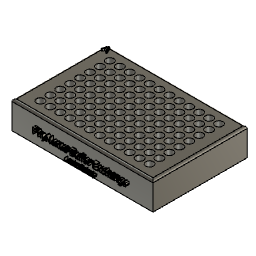
PhyNexus_Adapter v4 (Autodesk Fusion 360 design; units mm, degrees)
Autodesk Fusion 360 part; units mm, degrees
sketch "Sketch1" plane through (0, 0, 0) normal (0, 0, 1) x (1, 0, 0)
  line L0 (0, 0) -> (-127.8, 0)
  line L1 (-127.8, 0) -> (-127.8, 85.5)
  line L2 (-127.8, 85.5) -> (0, 85.5)
  line L3 (0, 85.5) -> (0, 0)
  dimension "d1" = 127.8
  dimension "d2" = 85.5
  constraint horizontal L0
  constraint vertical L1
  constraint horizontal L2
  constraint vertical L3
  constraint coincident L0.start L3.end
  measures "d1" distance of L0.start L0.end
  measures "d2" distance of L0.start L2.end
extrude "Extrude1" add sketch "Sketch1" along normal blind 25
sketch "Sketch2" plane through (0, 0, 25) normal (0, 0, 1) x (-1, 0, 0)
  line L0 (0, -85.5) -> (127.8, -85.5)
  line L1 (127.8, -85.5) -> (127.8, 0)
  line L2 (127.8, 0) -> (0, 0)
  line L3 (0, 0) -> (0, -85.5)
  circle A0 centre (113.4, -74.3) radius 3.5
  circle A1 centre (104.4, -74.3) radius 3.5
  circle A2 centre (95.4, -74.3) radius 3.5
  circle A3 centre (86.4, -74.3) radius 3.5
  circle A4 centre (77.4, -74.3) radius 3.5
  circle A5 centre (68.4, -74.3) radius 3.5
  circle A6 centre (59.4, -74.3) radius 3.5
  circle A7 centre (50.4, -74.3) radius 3.5
  circle A8 centre (41.4, -74.3) radius 3.5
  circle A9 centre (32.4, -74.3) radius 3.5
  circle A10 centre (23.4, -74.3) radius 3.5
  circle A11 centre (14.4, -74.3) radius 3.5
  circle A12 centre (113.4, -65.3) radius 3.5
  circle A13 centre (104.4, -65.3) radius 3.5
  circle A14 centre (95.4, -65.3) radius 3.5
  circle A15 centre (86.4, -65.3) radius 3.5
  circle A16 centre (77.4, -65.3) radius 3.5
  circle A17 centre (68.4, -65.3) radius 3.5
  circle A18 centre (59.4, -65.3) radius 3.5
  circle A19 centre (50.4, -65.3) radius 3.5
  circle A20 centre (41.4, -65.3) radius 3.5
  circle A21 centre (32.4, -65.3) radius 3.5
  circle A22 centre (23.4, -65.3) radius 3.5
  circle A23 centre (14.4, -65.3) radius 3.5
  circle A24 centre (113.4, -56.3) radius 3.5
  circle A25 centre (104.4, -56.3) radius 3.5
  circle A26 centre (95.4, -56.3) radius 3.5
  circle A27 centre (86.4, -56.3) radius 3.5
  circle A28 centre (77.4, -56.3) radius 3.5
  circle A29 centre (68.4, -56.3) radius 3.5
  circle A30 centre (59.4, -56.3) radius 3.5
  circle A31 centre (50.4, -56.3) radius 3.5
  circle A32 centre (41.4, -56.3) radius 3.5
  circle A33 centre (32.4, -56.3) radius 3.5
  circle A34 centre (23.4, -56.3) radius 3.5
  circle A35 centre (14.4, -56.3) radius 3.5
  circle A36 centre (113.4, -47.3) radius 3.5
  circle A37 centre (104.4, -47.3) radius 3.5
  circle A38 centre (95.4, -47.3) radius 3.5
  circle A39 centre (86.4, -47.3) radius 3.5
  circle A40 centre (77.4, -47.3) radius 3.5
  circle A41 centre (68.4, -47.3) radius 3.5
  circle A42 centre (59.4, -47.3) radius 3.5
  circle A43 centre (50.4, -47.3) radius 3.5
  circle A44 centre (41.4, -47.3) radius 3.5
  circle A45 centre (32.4, -47.3) radius 3.5
  circle A46 centre (23.4, -47.3) radius 3.5
  circle A47 centre (14.4, -47.3) radius 3.5
  circle A48 centre (113.4, -38.3) radius 3.5
  circle A49 centre (104.4, -38.3) radius 3.5
  circle A50 centre (95.4, -38.3) radius 3.5
  circle A51 centre (86.4, -38.3) radius 3.5
  circle A52 centre (77.4, -38.3) radius 3.5
  circle A53 centre (68.4, -38.3) radius 3.5
  circle A54 centre (59.4, -38.3) radius 3.5
  circle A55 centre (50.4, -38.3) radius 3.5
  circle A56 centre (41.4, -38.3) radius 3.5
  circle A57 centre (32.4, -38.3) radius 3.5
  circle A58 centre (23.4, -38.3) radius 3.5
  circle A59 centre (14.4, -38.3) radius 3.5
  circle A60 centre (113.4, -29.3) radius 3.5
  circle A61 centre (104.4, -29.3) radius 3.5
  circle A62 centre (95.4, -29.3) radius 3.5
  circle A63 centre (86.4, -29.3) radius 3.5
  circle A64 centre (77.4, -29.3) radius 3.5
  circle A65 centre (68.4, -29.3) radius 3.5
  circle A66 centre (59.4, -29.3) radius 3.5
  circle A67 centre (50.4, -29.3) radius 3.5
  circle A68 centre (41.4, -29.3) radius 3.5
  circle A69 centre (32.4, -29.3) radius 3.5
  circle A70 centre (23.4, -29.3) radius 3.5
  circle A71 centre (14.4, -29.3) radius 3.5
  circle A72 centre (113.4, -20.3) radius 3.5
  circle A73 centre (104.4, -20.3) radius 3.5
  circle A74 centre (95.4, -20.3) radius 3.5
  circle A75 centre (86.4, -20.3) radius 3.5
  circle A76 centre (77.4, -20.3) radius 3.5
  circle A77 centre (68.4, -20.3) radius 3.5
  circle A78 centre (59.4, -20.3) radius 3.5
  circle A79 centre (50.4, -20.3) radius 3.5
  circle A80 centre (41.4, -20.3) radius 3.5
  circle A81 centre (32.4, -20.3) radius 3.5
  circle A82 centre (23.4, -20.3) radius 3.5
  circle A83 centre (14.4, -20.3) radius 3.5
  circle A84 centre (113.4, -11.3) radius 3.5
  circle A85 centre (104.4, -11.3) radius 3.5
  circle A86 centre (95.4, -11.3) radius 3.5
  circle A87 centre (86.4, -11.3) radius 3.5
  circle A88 centre (77.4, -11.3) radius 3.5
  circle A89 centre (68.4, -11.3) radius 3.5
  circle A90 centre (59.4, -11.3) radius 3.5
  circle A91 centre (50.4, -11.3) radius 3.5
  circle A92 centre (41.4, -11.3) radius 3.5
  circle A93 centre (32.4, -11.3) radius 3.5
  circle A94 centre (23.4, -11.3) radius 3.5
  circle A95 centre (14.4, -11.3) radius 3.5
  dimension "d15" = 7
  dimension "d18" = -9
  dimension "d19" = 9
  measures "d15" diameter of A0
extrude "Extrude2" cut sketch "Sketch2" against normal blind 40 contours A0 | A1 | A2 | A3 | A4 | A5 | A6 | A7 | A8 | A9 | A10 | A11 | A12 | A13 | A14 | A15 | A16 | A17 | A18 | A19 | A20 | A21 | A22 | A23 | A24 | A25 | A26 | A27 | A28 | A29 | A30 | A31 | A32 | A33 | A34 | A35 | A36 | A37 | A38 | A39 | A40 | A41 | A42 | A43 | A44 | A45 | A46 | A47 | A48 | A49 | A50 | A51 | A52 | A53 | A54 | A55 | A56 | A57 | A58 | A59 | A60 | A61 | A62 | A63 | A64 | A65 | A66 | A67 | A68 | A69 | A70 | A71 | A72 | A73 | A74 | A75 | A76 | A77 | A78 | A79 | A80 | A81 | A82 | A83 | A84 | A85 | A86 | A87 | A88 | A89 | A90 | A91 | A92 | A93 | A94 | A95
sketch "Sketch4" plane through (0, 0, 0) normal (0, 0, -1) x (1, 0, 0)
  circle A0 centre (-95.4, -56.3) radius 3.5
  circle A1 centre (-86.4, -47.3) radius 3.5
  circle A2 centre (-68.4, -56.3) radius 3.5
  circle A3 centre (-86.4, -65.3) radius 3.5
  circle A4 centre (-68.4, -74.3) radius 3.5
  circle A5 centre (-104.4, -74.3) radius 3.5
  circle A6 centre (-86.4, -29.3) radius 3.5
  circle A7 centre (-68.4, -38.3) radius 3.5
  circle A8 centre (-104.4, -38.3) radius 3.5
  circle A9 centre (-86.4, -11.3) radius 3.5
  circle A10 centre (-68.4, -20.3) radius 3.5
  circle A11 centre (-104.4, -20.3) radius 3.5
  circle A12 centre (-32.4, -47.3) radius 3.5
  circle A13 centre (-14.4, -56.3) radius 3.5
  circle A14 centre (-59.4, -56.3) radius 3.5
  circle A15 centre (-32.4, -74.3) radius 3.5
  circle A16 centre (-14.4, -29.3) radius 3.5
  circle A17 centre (-50.4, -29.3) radius 3.5
  circle A18 centre (-23.4, -38.3) radius 3.5
  circle A19 centre (-23.4, -74.3) radius 3.5
  circle A20 centre (-50.4, -38.3) radius 3.5
  circle A21 centre (-32.4, -11.3) radius 3.5
  circle A22 centre (-14.4, -20.3) radius 3.5
  circle A23 centre (-50.4, -20.3) radius 3.5
  circle A24 centre (-41.4, -20.3) radius 3.5
  circle A25 centre (-59.4, -11.3) radius 3.5
  circle A26 centre (-23.4, -11.3) radius 3.5
  circle A27 centre (-41.4, -38.3) radius 3.5
  circle A28 centre (-86.4, -56.3) radius 3.5
  circle A29 centre (-14.4, -38.3) radius 3.5
  circle A30 centre (-41.4, -29.3) radius 3.5
  circle A31 centre (-59.4, -74.3) radius 3.5
  circle A32 centre (-50.4, -65.3) radius 3.5
  circle A33 centre (-50.4, -56.3) radius 3.5
  circle A34 centre (-59.4, -47.3) radius 3.5
  circle A35 centre (-23.4, -47.3) radius 3.5
  circle A36 centre (-95.4, -20.3) radius 3.5
  circle A37 centre (-113.4, -11.3) radius 3.5
  circle A38 centre (-77.4, -11.3) radius 3.5
  circle A39 centre (-95.4, -38.3) radius 3.5
  circle A40 centre (-113.4, -29.3) radius 3.5
  circle A41 centre (-77.4, -29.3) radius 3.5
  circle A42 centre (-95.4, -74.3) radius 3.5
  circle A43 centre (-113.4, -65.3) radius 3.5
  circle A44 centre (-77.4, -65.3) radius 3.5
  circle A45 centre (-113.4, -47.3) radius 3.5
  circle A46 centre (-77.4, -47.3) radius 3.5
  circle A47 centre (-14.4, -74.3) radius 3.5
  circle A48 centre (-59.4, -65.3) radius 3.5
  circle A49 centre (-95.4, -47.3) radius 3.5
  circle A50 centre (-113.4, -56.3) radius 3.5
  circle A51 centre (-95.4, -65.3) radius 3.5
  circle A52 centre (-77.4, -74.3) radius 3.5
  circle A53 centre (-113.4, -74.3) radius 3.5
  circle A54 centre (-95.4, -29.3) radius 3.5
  circle A55 centre (-77.4, -38.3) radius 3.5
  circle A56 centre (-113.4, -38.3) radius 3.5
  circle A57 centre (-95.4, -11.3) radius 3.5
  circle A58 centre (-77.4, -20.3) radius 3.5
  circle A59 centre (-113.4, -20.3) radius 3.5
  circle A60 centre (-41.4, -47.3) radius 3.5
  circle A61 centre (-23.4, -56.3) radius 3.5
  circle A62 centre (-14.4, -65.3) radius 3.5
  circle A63 centre (-41.4, -74.3) radius 3.5
  circle A64 centre (-23.4, -29.3) radius 3.5
  circle A65 centre (-59.4, -20.3) radius 3.5
  circle A66 centre (-32.4, -38.3) radius 3.5
  circle A67 centre (-23.4, -65.3) radius 3.5
  circle A68 centre (-59.4, -38.3) radius 3.5
  circle A69 centre (-41.4, -11.3) radius 3.5
  circle A70 centre (-23.4, -20.3) radius 3.5
  circle A71 centre (-104.4, -56.3) radius 3.5
  circle A72 centre (-32.4, -20.3) radius 3.5
  circle A73 centre (-50.4, -11.3) radius 3.5
  circle A74 centre (-14.4, -11.3) radius 3.5
  circle A75 centre (-41.4, -56.3) radius 3.5
  circle A76 centre (-77.4, -56.3) radius 3.5
  circle A77 centre (-59.4, -29.3) radius 3.5
  circle A78 centre (-32.4, -29.3) radius 3.5
  circle A79 centre (-50.4, -74.3) radius 3.5
  circle A80 centre (-41.4, -65.3) radius 3.5
  circle A81 centre (-32.4, -56.3) radius 3.5
  circle A82 centre (-50.4, -47.3) radius 3.5
  circle A83 centre (-14.4, -47.3) radius 3.5
  circle A84 centre (-86.4, -20.3) radius 3.5
  circle A85 centre (-104.4, -11.3) radius 3.5
  circle A86 centre (-68.4, -11.3) radius 3.5
  circle A87 centre (-86.4, -38.3) radius 3.5
  circle A88 centre (-104.4, -29.3) radius 3.5
  circle A89 centre (-68.4, -29.3) radius 3.5
  circle A90 centre (-86.4, -74.3) radius 3.5
  circle A91 centre (-104.4, -65.3) radius 3.5
  circle A92 centre (-68.4, -65.3) radius 3.5
  circle A93 centre (-104.4, -47.3) radius 3.5
  circle A94 centre (-68.4, -47.3) radius 3.5
  circle A95 centre (-32.4, -65.3) radius 3.5
  line L0 (-127.8, -85.5) -> (0, -85.5)
  line L1 (0, -85.5) -> (0, 0)
  line L2 (0, 0) -> (-127.8, 0)
  line L3 (-127.8, 0) -> (-127.8, -85.5)
  line L4 (-126.8, -1) -> (-1, -1)
  line L5 (-1, -1) -> (-1, -84.5)
  line L6 (-1, -84.5) -> (-126.8, -84.5)
  line L7 (-126.8, -84.5) -> (-126.8, -1)
  dimension "d26" = 1
  dimension "d27" = 1
  dimension "d28" = 1
  dimension "d29" = 1
  constraint horizontal L4
  constraint vertical L5
  constraint horizontal L6
  constraint vertical L7
  measures "d26" distance of L2 L4
  measures "d27" distance of L3 L7
  measures "d28" distance of L0 L6
  measures "d29" distance of L1 L5
extrude "Extrude3" cut sketch "Sketch4" against normal blind 5 contours L4 L5 L6 L7
sketch "Sketch5" plane through (0, 0, 0) normal (0, -1, 0) x (1, 0, 0)
  line L0 (-127.8, 0) -> (0, 0)
  line L1 (0, 0) -> (0, 25)
  line L2 (0, 25) -> (-127.8, 25)
  line L3 (-127.8, 25) -> (-127.8, 0)
  line L4 (-127.8, 9) -> (0, 9) construction
  line L5 (0, 9) -> (0, 16) construction
  line L6 (0, 16) -> (-127.8, 16) construction
  line L7 (-127.8, 16) -> (-127.8, 9) construction
  line L8 (-127.8, 0.6321) -> (0, 0.6321) construction
  line L9 (0, 0.6321) -> (0, 7.6321) construction
  line L10 (0, 7.6321) -> (-127.8, 7.6321) construction
  line L11 (-127.8, 7.6321) -> (-127.8, 0.6321) construction
  dimension "d32" = 5
  dimension "d33" = 9
  dimension "d34" = 9
  dimension "d35" = 2.5
  text T0 "PhyNexus Buffer Exchange" font "Arial" height 5 align centre middle in box 127.8 x 7 at (-127.8, 9) x (1, 0) y (0, 1) spacing 1
  text T1 "London Biofoudry" font "Arial" height 2.5 align centre middle in box 127.8 x 7 at (-127.8, 0.6321) x (1, 0) y (0, 1) spacing 1
  constraint coincident L3
  constraint coincident L1
  constraint parallel L2 L6
  measures "d33" distance of L2 L6
  measures "d34" distance of L0 L4
extrude "Extrude4" add sketch "Sketch5" along normal blind 3 text T1 T0
sketch "Sketch6" plane through (0, 0, 25) normal (0, 0, 1) x (-1, 0, 0)
  circle A0 centre (95.4, -56.3) radius 3.5
  circle A1 centre (86.4, -47.3) radius 3.5
  circle A2 centre (68.4, -56.3) radius 3.5
  circle A3 centre (86.4, -65.3) radius 3.5
  circle A4 centre (68.4, -74.3) radius 3.5
  circle A5 centre (104.4, -74.3) radius 3.5
  circle A6 centre (86.4, -29.3) radius 3.5
  circle A7 centre (68.4, -38.3) radius 3.5
  circle A8 centre (104.4, -38.3) radius 3.5
  circle A9 centre (86.4, -11.3) radius 3.5
  circle A10 centre (68.4, -20.3) radius 3.5
  circle A11 centre (104.4, -20.3) radius 3.5
  circle A12 centre (32.4, -47.3) radius 3.5
  circle A13 centre (14.4, -56.3) radius 3.5
  circle A14 centre (59.4, -56.3) radius 3.5
  circle A15 centre (32.4, -74.3) radius 3.5
  circle A16 centre (14.4, -29.3) radius 3.5
  circle A17 centre (50.4, -29.3) radius 3.5
  circle A18 centre (23.4, -38.3) radius 3.5
  circle A19 centre (23.4, -74.3) radius 3.5
  circle A20 centre (50.4, -38.3) radius 3.5
  circle A21 centre (32.4, -11.3) radius 3.5
  circle A22 centre (14.4, -20.3) radius 3.5
  circle A23 centre (50.4, -20.3) radius 3.5
  circle A24 centre (41.4, -20.3) radius 3.5
  circle A25 centre (59.4, -11.3) radius 3.5
  circle A26 centre (23.4, -11.3) radius 3.5
  circle A27 centre (41.4, -38.3) radius 3.5
  circle A28 centre (86.4, -56.3) radius 3.5
  circle A29 centre (14.4, -38.3) radius 3.5
  circle A30 centre (41.4, -29.3) radius 3.5
  circle A31 centre (59.4, -74.3) radius 3.5
  circle A32 centre (50.4, -65.3) radius 3.5
  circle A33 centre (50.4, -56.3) radius 3.5
  circle A34 centre (59.4, -47.3) radius 3.5
  circle A35 centre (23.4, -47.3) radius 3.5
  circle A36 centre (95.4, -20.3) radius 3.5
  circle A37 centre (113.4, -11.3) radius 3.5
  circle A38 centre (77.4, -11.3) radius 3.5
  circle A39 centre (95.4, -38.3) radius 3.5
  circle A40 centre (113.4, -29.3) radius 3.5
  circle A41 centre (77.4, -29.3) radius 3.5
  circle A42 centre (95.4, -74.3) radius 3.5
  circle A43 centre (113.4, -65.3) radius 3.5
  circle A44 centre (77.4, -65.3) radius 3.5
  circle A45 centre (113.4, -47.3) radius 3.5
  circle A46 centre (77.4, -47.3) radius 3.5
  circle A47 centre (14.4, -74.3) radius 3.5
  circle A48 centre (59.4, -65.3) radius 3.5
  circle A49 centre (95.4, -47.3) radius 3.5
  circle A50 centre (113.4, -56.3) radius 3.5
  circle A51 centre (95.4, -65.3) radius 3.5
  circle A52 centre (77.4, -74.3) radius 3.5
  circle A53 centre (113.4, -74.3) radius 3.5
  circle A54 centre (95.4, -29.3) radius 3.5
  circle A55 centre (77.4, -38.3) radius 3.5
  circle A56 centre (113.4, -38.3) radius 3.5
  circle A57 centre (95.4, -11.3) radius 3.5
  circle A58 centre (77.4, -20.3) radius 3.5
  circle A59 centre (113.4, -20.3) radius 3.5
  circle A60 centre (41.4, -47.3) radius 3.5
  circle A61 centre (23.4, -56.3) radius 3.5
  circle A62 centre (14.4, -65.3) radius 3.5
  circle A63 centre (41.4, -74.3) radius 3.5
  circle A64 centre (23.4, -29.3) radius 3.5
  circle A65 centre (59.4, -20.3) radius 3.5
  circle A66 centre (32.4, -38.3) radius 3.5
  circle A67 centre (23.4, -65.3) radius 3.5
  circle A68 centre (59.4, -38.3) radius 3.5
  circle A69 centre (41.4, -11.3) radius 3.5
  circle A70 centre (23.4, -20.3) radius 3.5
  circle A71 centre (104.4, -56.3) radius 3.5
  circle A72 centre (32.4, -20.3) radius 3.5
  circle A73 centre (50.4, -11.3) radius 3.5
  circle A74 centre (14.4, -11.3) radius 3.5
  circle A75 centre (41.4, -56.3) radius 3.5
  circle A76 centre (77.4, -56.3) radius 3.5
  circle A77 centre (59.4, -29.3) radius 3.5
  circle A78 centre (32.4, -29.3) radius 3.5
  circle A79 centre (50.4, -74.3) radius 3.5
  circle A80 centre (41.4, -65.3) radius 3.5
  circle A81 centre (32.4, -56.3) radius 3.5
  circle A82 centre (50.4, -47.3) radius 3.5
  circle A83 centre (14.4, -47.3) radius 3.5
  circle A84 centre (86.4, -20.3) radius 3.5
  circle A85 centre (104.4, -11.3) radius 3.5
  circle A86 centre (68.4, -11.3) radius 3.5
  circle A87 centre (86.4, -38.3) radius 3.5
  circle A88 centre (104.4, -29.3) radius 3.5
  circle A89 centre (68.4, -29.3) radius 3.5
  circle A90 centre (86.4, -74.3) radius 3.5
  circle A91 centre (104.4, -65.3) radius 3.5
  circle A92 centre (68.4, -65.3) radius 3.5
  circle A93 centre (104.4, -47.3) radius 3.5
  circle A94 centre (68.4, -47.3) radius 3.5
  circle A95 centre (32.4, -65.3) radius 3.5
  line L0 (0, -85.5) -> (127.8, -85.5)
  line L1 (127.8, -85.5) -> (127.8, 0)
  line L2 (127.8, 0) -> (0, 0)
  line L3 (0, 0) -> (0, -85.5)
  line L4 (126.5308, -3.4707) -> (118.8988, -3.4707) construction
  line L5 (118.8988, -3.4707) -> (118.8988, -83.2455) construction
  line L6 (118.8988, -83.2455) -> (126.5308, -83.2455) construction
  line L7 (126.5308, -83.2455) -> (126.5308, -3.4707) construction
  dimension "d38" = 5
  text T0 "A" font "Arial" height 5 align centre top in box 7.6319 x 79.7748 at (126.5308, -3.4707) x (-1, 0) y (0, -1) spacing 1.03
  constraint parallel L1 L7
extrude "Extrude5" add sketch "Sketch6" along normal blind 2 text T0
fillet "Fillet1" radius 2 4 edges at (-63.9, 0, 25) (-127.8, 42.75, 25) (-63.9, 85.5, 25) (0, 42.75, 25)
